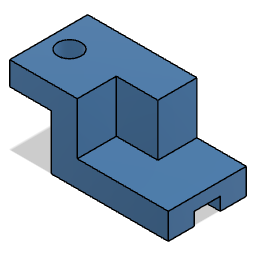
3d02 v1 (Autodesk Fusion 360 design; units mm, degrees)
Autodesk Fusion 360 part; units mm, degrees
sketch "Sketch1" plane through (0, 0, 0) normal (0, 1, 0) x (1, 0, 0)
  line L0 (0, 0) -> (61, 0)
  line L1 (61, 0) -> (61, -30)
  line L2 (61, -30) -> (0, -30)
  line L3 (0, -30) -> (0, 0)
  dimension "d1" = 61
  dimension "d2" = 30
  constraint horizontal L0
  constraint vertical L1
  constraint horizontal L2
  constraint vertical L3
  constraint coincident L0.start L3.end
  measures "d1" distance of L0.start L0.end
  measures "d2" distance of L0.start L2.end
extrude "Extrude1" add sketch "Sketch1" along normal blind 10
sketch "Sketch2" plane through (0, 10, 0) normal (0, 1, 0) x (-1, 0, 0)
  line L0 (0, 30) -> (-61, 30)
  line L1 (-61, 30) -> (-61, 0)
  line L2 (-61, 0) -> (0, 0)
  line L3 (0, 0) -> (0, 30)
  line L4 (0, 0) -> (-26, 0)
  line L5 (-26, 0) -> (-26, 30)
  line L6 (-26, 30) -> (0, 30)
  line L7 (0, 30) -> (0, 0)
  dimension "d5" = 26
  constraint horizontal L4
  constraint vertical L5
  constraint horizontal L6
  constraint vertical L7
  constraint coincident L2.end L3.start
  measures "d5" distance of L2.end L4.end
extrude "Extrude2" add sketch "Sketch2" along normal blind 20 contours L0 L2 L3 L4 L5 L6 L7
sketch "Sketch3" plane through (0, 30, 0) normal (0, 1, 0) x (-1, 0, 0)
  line L0 (0, 30) -> (-26, 30)
  line L1 (-26, 30) -> (-26, 0)
  line L2 (-26, 0) -> (0, 0)
  line L3 (0, 0) -> (0, 30)
  line L4 (-26, 0) -> (-42, 0)
  line L5 (-42, 0) -> (-42, 15)
  line L6 (-42, 15) -> (-26, 15)
  line L7 (-26, 15) -> (-26, 0)
  dimension "d8" = 16
  dimension "d9" = 15
  constraint horizontal L4
  constraint vertical L5
  constraint horizontal L6
  constraint vertical L7
  constraint coincident L1.end L2.start
  measures "d8" distance of L1.end L4.end
  measures "d9" distance of L1.end L6.end
extrude "Extrude3" add sketch "Sketch3" against normal up to surface (20 mm away) contours L1 L4 L5 L6 L7
sketch "Sketch4" plane through (0, 0, 30) normal (0, 0, 1) x (1, 0, 0)
  line L0 (0, 0) -> (61, 0)
  line L1 (61, 0) -> (61, 10)
  line L2 (61, 10) -> (26, 10)
  line L3 (26, 10) -> (26, 30)
  line L4 (26, 30) -> (0, 30)
  line L5 (0, 30) -> (0, 0)
  line L6 (0, 0) -> (16, 0)
  line L7 (16, 0) -> (16, 21)
  line L8 (16, 21) -> (0, 21)
  line L9 (0, 21) -> (0, 0)
  dimension "d12" = 16
  dimension "d13" = 21
  constraint horizontal L6
  constraint vertical L7
  constraint horizontal L8
  constraint vertical L9
  constraint coincident L0.start L5.end
  measures "d12" distance of L0.start L6.end
  measures "d13" distance of L0.start L8.end
extrude "Extrude4" cut sketch "Sketch4" against normal blind 30 contours L0 L5 L6 L7 L8 L9
sketch "Sketch5" plane through (0, 30, 0) normal (0, 1, 0) x (-1, 0, 0)
  line L0 (0, 30) -> (-26, 30)
  line L1 (-26, 30) -> (-26, 15)
  line L2 (-26, 15) -> (-42, 15)
  line L3 (-42, 15) -> (-42, 0)
  line L4 (-42, 0) -> (0, 0)
  line L5 (0, 0) -> (0, 30)
  line L6 (28.1028, 15) -> (-28.1028, 15) construction
  circle A0 centre (-8, 15) radius 4.5
  dimension "d16" = 9
  dimension "d17" = 8
  constraint horizontal L6
  constraint midpoint L5 L6
  constraint coincident L6 A0.centre
  measures "d16" diameter of A0
  measures "d17" horizontal distance of L4.end A0.centre
extrude "Extrude5" cut sketch "Sketch5" against normal blind 9 contours A0
sketch "Sketch6" plane through (61, 0, 0) normal (1, 0, 0) x (0, 0, -1)
  line L0 (-30, 0) -> (0, 0)
  line L1 (0, 0) -> (0, 10)
  line L2 (0, 10) -> (-30, 10)
  line L3 (-30, 10) -> (-30, 0)
  line L4 (-20, 0) -> (-20, 5)
  line L5 (-20, 5) -> (-10, 5)
  line L6 (-10, 5) -> (-10, 0)
  dimension "d20" = 10
  dimension "d21" = 5
  dimension "d22" = 5
  dimension "d23" = 10
  constraint vertical L4
  constraint perpendicular L4 L5
  constraint perpendicular L5 L6
  constraint horizontal L0.end L4.start
  measures "d20" distance of L4.end L5.end
  measures "d21" distance of L4.start L4.end
  measures "d22" distance of L5.end L6.end
  measures "d23" horizontal distance of L0.start L4.start
extrude "Extrude6" cut sketch "Sketch6" against normal blind 45 contours L0 L4 L5 L6
